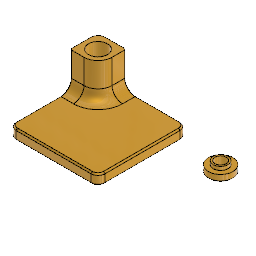
Board_post v6 (Autodesk Fusion 360 design; units mm, degrees)
Autodesk Fusion 360 part; units mm, degrees
sketch "Sketch1" plane through (0, 0, 0) normal (0, 0, 1) x (1, 0, 0)
  circle A0 centre (0, 0) radius 2.7
  circle A1 centre (0, 0) radius 4
  line L0 (4, -4) -> (-4, -4)
  line L1 (-4, -4) -> (-4, 4)
  line L2 (-4, 4) -> (4, 4)
  line L3 (4, 4) -> (4, -4)
  line L4 (4, -4) -> (-4, 4) construction
  line L5 (-4, -4) -> (4, 4) construction
  circle A2 centre (35, 0) radius 1.6
  circle A3 centre (35, 0) radius 2.1
  circle A4 centre (35, 0) radius 3.5
  line L6 (-4, 4) -> (21.4, 4)
  line L7 (21.4, 4) -> (21.4, -21.4)
  line L8 (21.4, -21.4) -> (-4, -21.4)
  line L9 (-4, -21.4) -> (-4, 4)
  dimension "d3" = 5.4
  dimension "d4" = 8
  dimension "d15" = 3.2
  dimension "d16" = 4.2
  dimension "d17" = 7
  dimension "d25" = 25.4
  dimension "d26" = 25.4
  constraint coincident A0.centre A1.centre
  constraint perpendicular L0 L1
  constraint parallel L0 L2
  constraint parallel L1 L3
  constraint horizontal L0
  constraint coincident L4 A0.centre
  constraint coincident L5 A0.centre
  constraint tangent A1 L1
  constraint concentric A2 A3
  constraint concentric A3 A4
  constraint horizontal L6
  constraint vertical L7
  constraint horizontal L8
  constraint vertical L9
  measures "d3" diameter of A0
  measures "d4" diameter of A1
  measures "d15" diameter of A2
  measures "d16" diameter of A3
  measures "d17" diameter of A4
  measures "d25" distance of L1.end L6.end
  measures "d26" distance of L1.end L8.end
extrude "Extrude1" add sketch "Sketch1" along normal blind 3 contours A0 | A1 | A1 L0 L3 | A1 L2 L3 L6 | L0 L3 L6 L7 L8 L9 | A1 L1 L2 L6 L9 | A1 L0 L1 L9 makes body 1
extrude "Extrude2" add sketch "Sketch1" along normal blind 10 from surface at 3 contours A0 | A1 | A1 L2 L3 L6 | A1 L1 L2 L6 L9 | A1 L0 L1 L9 bodies 1
extrude "Extrude3" cut sketch "Sketch1" against normal blind 8 from surface at 13 contours A0 bodies 1
fillet "Fillet2" radius 2 4 edges at (-4, 4, 6.5) (21.4, 4, 1.5) (21.4, -21.4, 1.5) (-4, -21.4, 1.5) on bodies 1
fillet "Fillet3" radius 3 3 edges at (4, 2, 3) (2.8284, -2.8284, 3) (-2, -4, 3) on bodies 1
chamfer "Chamfer4" distance 0.4 angle 45 8 edges at (20.8142, -20.8142, 0) (8.7, -21.4, 0) (-3.4142, -20.8142, 0) (-4, -8.7, 0) (-3.4142, 3.4142, 0) (8.7, 4, 0) (20.8142, 3.4142, 0) (21.4, -8.7, 0) on bodies 1
chamfer "Chamfer6" distance 0.4 angle 45 11 edges at (4, 4, 9.5) (4.8787, 4, 3.8787) (13.2, 4, 3) (20.8142, 3.4142, 3) (21.4, -8.7, 3) (20.8142, -20.8142, 3) (8.7, -21.4, 3) (-3.4142, -20.8142, 3) (-4, -13.2, 3) (-4, -4.8787, 3.8787) (-4, -4, 9.5) on bodies 1
extrude "Extrude4" add sketch "Sketch1" along normal blind 2 separate body contours A3 | A4 makes body 2
extrude "Extrude5" add sketch "Sketch1" along normal blind 1 from surface at 2 contours A3 bodies 2
chamfer "Chamfer2" distance 0.4 angle 45 1 edges at (31.7369, -1.2657, 0) on bodies 2
